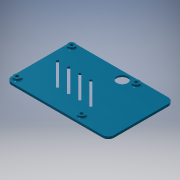
# Autodesk Inventor part: case_bottom
Saved by Autodesk Inventor 2019 (Build 230136000, 136)
## iProperties
Created: 2020-03-30
Part Number: case_bottom
Material: 1.4301
Document SubType Name: Modellieren
Designer: saa
Manufacturer: Standard
Standards Organization: Custom
Density: 7.86 g/cm^3
Appearance: RAL 5001 Grünblau
Author: saa
Autodesk Inventor part; units mm, degrees
ref_plane "YZ Ebene" through (0, 0, 0) normal (1, 0, 0) x (0, 1, 0)
ref_plane "XZ Ebene" through (0, 0, 0) normal (0, 1, 0) x (-1, 0, 0)
ref_plane "XY Ebene" through (0, 0, 0) normal (0, 0, 1) x (1, 0, 0)
sketch "Skizze5" plane through (0, 0, 0) normal (0, 0, 1) x (1, 0, 0)
  line L0 (0, 0) -> (92, 0)
  line L1 (92, 0) -> (92, 59)
  line L2 (92, 59) -> (0, 59)
  line L3 (0, 59) -> (0, 0)
  dimension "d33" = 59
  dimension "d34" = 92
  constraints: 8 end point, 2 parallel, 1 horizontal, 1 perpendicular
  measures "d33" distance of L2.end L0.start
  measures "d34" distance of L0.start L0.end
extrude "Extrusion5" add sketch "Skizze5" along normal blind 2
fillet "Rundung2" radius 5 4 edges at (0, 0, 1) (92, 0, 1) (92, 59, 1) (0, 59, 1)
sketch "Skizze6" plane through (0, 0, 2) normal (0, 0, 1) x (1, 0, 0)
  line L0 (6.0469, 57.9713) -> (80.9531, 57.9713) construction
  line L1 (86, 52.9244) -> (86, 7.0182) construction
  line L2 (80.9531, 1.9713) -> (6.0469, 1.9713) construction
  line L3 (1, 7.0182) -> (1, 52.9244) construction
  arc A0 (6.0469, 57.9713) -> (1, 52.9244) centre (6.0469, 52.9244) ccw construction
  arc A1 (86, 52.9244) -> (80.9531, 57.9713) centre (80.9531, 52.9244) ccw construction
  arc A2 (80.9531, 1.9713) -> (86, 7.0182) centre (80.9531, 7.0182) ccw
  arc A3 (1, 7.0182) -> (6.0469, 1.9713) centre (6.0469, 7.0182) ccw construction
  line L4 (0, 51.6837) -> (0, 8.2589)
  line L5 (0, 29.9713) -> (94.8854, 29.9713) construction
  circle A4 centre (4.5, 54.4713) radius 3
  circle A5 centre (4.5, 5.4713) radius 3
  circle A6 centre (62.5, 54.4713) radius 3
  line L6 (4.5, 54.4713) -> (62.5, 54.4713) construction
  line L7 (62.5, 54.4713) -> (62.5, 5.4713) construction
  line L8 (62.5, 5.4713) -> (4.5, 5.4713) construction
  line L9 (4.5, 5.4713) -> (4.5, 54.4713) construction
  circle A7 centre (62.5, 5.4713) radius 3
  line L10 (0, 54) -> (0, 5) projected
  point P0 (0, 0)
  point P1 (-5, -59)
  dimension "d38" = 85
  dimension "d39" = 56
  dimension "d40" = 1
  dimension "d41" = 6
  dimension "d42" = 3.5
  dimension "d43" = 3.5
  dimension "d44" = 6
  dimension "d45" = 3.5
  dimension "d46" = 3.5
  dimension "d47" = 6
  dimension "d48" = 6
  dimension "d49" = 58
  dimension "d50" = 3.5
  constraints: 20 end point, 8 centre point, 8 point on circle, 8 tangent, 4 parallel, 3 equal radius, 3 horizontal, 2 coincident, 2 perpendicular, 1 collinear, 1 midpoint, 1 other
  measures "d38" distance between parallel lines of L1 L3
  measures "d39" distance between parallel lines of L2 L0
  measures "d40" distance between parallel lines of L4 L3
  measures "d41" diameter of A4
  measures "d42" distance from line of L3 L9.end
  measures "d43" distance from line of L0 L9.end
  measures "d44" diameter of A5
  measures "d45" distance from line of L2 A5.centre
  measures "d46" distance from line of L3 A5.centre
  measures "d47" diameter of A6
  measures "d48" diameter of A7
  measures "d49" distance of L9.end L7.start
  measures "d50" distance between parallel lines of L2 L8
extrude "Extrusion6" add sketch "Skizze6" along normal blind 2
sketch "Skizze7" plane through (0, 0, 2) normal (0, 0, 1) x (1, 0, 0)
  circle A0 centre (62.5, 54.4713) radius 3 projected
  point P0 (0, 0)
  point P1 (52.5, 51.9713)
  dimension "d53" = 10
  dimension "d54" = 2.5
  measures "d53" horizontal distance of A0.centre point (52.5, 51.971)
  measures "d54" vertical distance of point (52.5, 51.971) A0.centre
hole "Antenne" at (52.5, 51.9713, 2) direction (0, 0, -1) diameter 10 depth 8.5 tip angle 118
fillet "Rundung3" radius 1 1 edges at (52.5, 56.9713, 0)
fillet "Rundung4" radius 1 4 edges at (59.5, 54.4713, 2) (1.5, 54.4713, 2) (1.5, 5.4713, 2) (59.5, 5.4713, 2)
sketch "Skizze8" plane through (0, 0, 0) normal (0, 0, -1) x (-1, 0, 0)
  circle A0 centre (-4.5, 5.4713) radius 3 construction
  circle A1 centre (-4.5, 54.4713) radius 3 construction
  circle A2 centre (-62.5, 54.4713) radius 3 construction
  circle A3 centre (-62.5, 5.4713) radius 3 construction
  point P0 (0, 0)
hole "Bohrung2" at (4.5, 54.4713, 0) at (4.5, 5.4713, 0) at (62.5, 5.4713, 0) at (62.5, 54.4713, 0) direction (0, 0, 1) diameter 2.75 depth 8 tip angle 118 counterbore diameter 5.5 counterbore depth 1.35
sketch "Skizze9" plane through (0, 0, 0) normal (0, 0, -1) x (-1, 0, 0)
  line L0 (-8.9971, 38.7452) -> (-7.5829, 37.331)
  line L1 (-7.5829, 37.331) -> (-28.7961, 16.1178)
  line L2 (-28.7961, 16.1178) -> (-30.2103, 17.532)
  line L3 (-30.2103, 17.532) -> (-8.9971, 38.7452)
  line L4 (-5, 0) -> (-87, 0) projected
  point P0 (0, 0)
  dimension "d72" = 2
  dimension "d74" = 45
  dimension "d75" = 30
  constraints: 8 end point, 2 parallel, 1 perpendicular
  measures "d72" distance between parallel lines of L3 L1
  measures "d74" angle of L4 L1
  measures "d75" distance of L0.end L1.end
extrude "Extrusion7" cut sketch "Skizze9" against normal blind 2
fillet "Rundung5" radius 0.5 4 edges at (8.9971, 38.7452, 1) (7.5829, 37.331, 1) (30.2103, 17.532, 1) (28.7961, 16.1178, 1)
fillet "Rundung6" radius 1 4 edges at (30.0032, 17.532, 0) (19.6037, 28.1386, 0) (8.9971, 38.5381, 0) (18.1895, 26.7244, 0)
pattern_linear "Rechteckige Anordnung1" count 4 spacing 10 along (1, 0, 0) of "Rundung6", "Extrusion7", "Rundung5"
